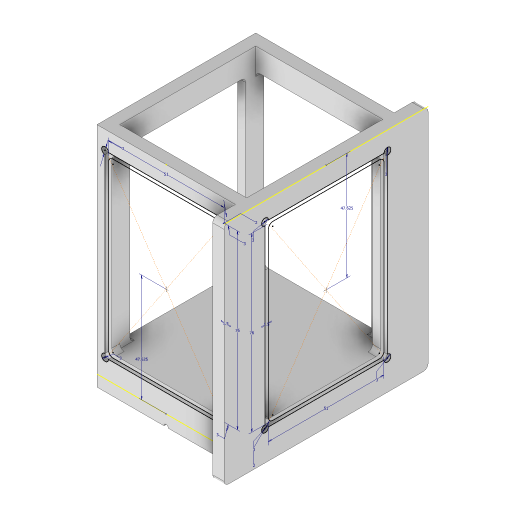
# Autodesk Inventor part: cuvette-w70mm-slide50x75mm-v1
Saved by Autodesk Inventor 2023 (Build 270158000, 158)
## iProperties
Created: 2025-09-30
Part Number: cuvette-w70mm-slide50x75mm-v1
Material: Generic
Document SubType Name: Modeling
Designer: N.Vladimirov
Density: 1 g/cm^3
Appearance: Default
Author: N.Vladimirov
Autodesk Inventor part; units mm, degrees
ref_plane "YZ Plane" through (0, 0, 0) normal (1, 0, 0) x (0, 1, 0)
ref_plane "XZ Plane" through (0, 0, 0) normal (0, 1, 0) x (-1, 0, 0)
ref_plane "XY Plane" through (0, 0, 0) normal (0, 0, 1) x (1, 0, 0)
sketch "Sketch1" plane through (0, 0, 0) normal (0, 0, 1) x (1, 0, 0)
  line L0 (30.5, -35) -> (-30.5, -35)
  line L1 (-30.5, -35) -> (-30.5, 35)
  line L2 (-30.5, 35) -> (30.5, 35)
  line L3 (30.5, 35) -> (30.5, -35)
  line L4 (30.5, -35) -> (-30.5, 35) construction
  line L5 (-30.5, -35) -> (30.5, 35) construction
  point P0 (0, 0)
  dimension "d0" = 61
  dimension "d1" = 70
  constraints: 12 end point, 2 midpoint, 2 parallel, 1 horizontal, 1 perpendicular
  measures "d0" distance of L1.end L2.end
  measures "d1" distance of L0.end L1.end
extrude "Extrusion1" add sketch "Sketch1" along normal blind 95.25
sketch "Sketch2" plane through (30.5, -35, 0) normal (1, 0, 0) x (0, 0, -1)
  line L0 (0, 0) -> (0, 70) projected
  line L1 (0, 70) -> (-95.25, 70) projected
  line L2 (-95.25, 0) -> (-95.25, 70) projected
  line L3 (0, 0) -> (-95.25, 0) projected
  line L4 (0, 70) -> (-95.25, 70) projected
  line L5 (-95.25, 70) -> (0, 70)
  line L6 (0, 70) -> (0, 80)
  line L7 (0, 80) -> (-95.25, 80)
  line L8 (-95.25, 80) -> (-95.25, 70)
  line L9 (-95.25, 70) -> (-95.25, 0) projected
  line L10 (-95.25, 0) -> (0, 0)
  line L11 (0, 0) -> (0, -10)
  line L12 (0, -10) -> (-95.25, -10)
  line L13 (-95.25, -10) -> (-95.25, 0)
  point P0 (0, 35)
  dimension "d4" = 10
  dimension "d5" = 10
  constraints: 16 end point, 4 parallel, 2 horizontal, 2 perpendicular, 1 point on line
  measures "d4" distance of L6.end L5.end
  measures "d5" distance of L10.end L11.end
extrude "Extrusion2" add sketch "Sketch2" along normal blind 5
sketch "Sketch3" plane through (35.5, -35, 0) normal (1, 0, 0) x (0, 0, -1)
  line L0 (0, -10) -> (0, 80) projected
  line L1 (-11.625, 9.5) -> (-83.625, 9.5)
  line L2 (-85.625, 11.5) -> (-85.625, 58.5)
  line L3 (-83.625, 60.5) -> (-11.625, 60.5)
  line L4 (-9.625, 58.5) -> (-9.625, 11.5)
  line L5 (-9.625, 9.5) -> (-85.625, 60.5) construction
  line L6 (-85.625, 9.5) -> (-9.625, 60.5) construction
  line L7 (-9.625, 62) -> (-85.625, 62)
  line L8 (-87.125, 60.5) -> (-87.125, 9.5)
  line L9 (-85.625, 8) -> (-9.625, 8)
  line L10 (-8.125, 9.5) -> (-8.125, 60.5)
  arc A0 (-85.625, 62) -> (-87.125, 60.5) centre (-87.125, 62) ccw
  arc A1 (-8.125, 60.5) -> (-9.625, 62) centre (-8.125, 62) ccw
  arc A2 (-87.125, 9.5) -> (-85.625, 8) centre (-87.125, 8) ccw
  arc A3 (-9.625, 8) -> (-8.125, 9.5) centre (-8.125, 8) ccw
  arc A4 (-83.625, 60.5) -> (-85.625, 58.5) centre (-83.625, 58.5) ccw
  arc A5 (-85.625, 11.5) -> (-83.625, 9.5) centre (-83.625, 11.5) ccw
  arc A6 (-9.625, 58.5) -> (-11.625, 60.5) centre (-11.625, 58.5) ccw
  arc A7 (-11.625, 9.5) -> (-9.625, 11.5) centre (-11.625, 11.5) ccw
  point P0 (0, 35)
  point P1 (-47.625, 35)
  point P2 (0, 35)
  dimension "d8" = 47.625
  dimension "d9" = 76
  dimension "d10" = 51
  dimension "d11" = 1.5
  dimension "d12" = 3
  dimension "d13" = 3
  dimension "d14" = 3
  dimension "d15" = 3
  dimension "d16" = 2
  constraints: 20 end point, 16 point on circle, 8 centre point, 8 point on line, 8 tangent, 4 parallel, 3 equal radius, 3 midpoint, 2 perpendicular, 1 horizontal
  measures "d8" distance of point (0, 35) point (-47.625, 35)
  measures "d9" distance of L5.end L6.end
  measures "d10" distance of L6.start L5.end
  measures "d11" distance between parallel lines of L3 L7
  measures "d12" diameter of A0
  measures "d13" diameter of A1
  measures "d14" diameter of A2
  measures "d15" diameter of A3
  measures "d16" radius of A4
extrude "Extrusion3" cut sketch "Sketch3" against normal through all contours L1 A5 L2 A4 L3 A6 L4 A7
extrude "Extrusion4" cut sketch "Sketch3" against normal blind 1.5 contours L1 A5 L2 A4 L3 A6 L4 A7 | A1 L10 A3 L9 A2 L8 A0 L7
sketch "Sketch4" plane through (-30.5, -35, 0) normal (-1, 0, 0) x (0, 0, 1)
  arc A0 (9.625, 62) -> (8.125, 60.5) centre (8.125, 62) ccw projected
  line L0 (8.125, 60.5) -> (8.125, 9.5) projected
  line L1 (85.625, 62) -> (9.625, 62) projected
  arc A1 (8.125, 9.5) -> (9.625, 8) centre (8.125, 8) ccw projected
  line L2 (9.625, 8) -> (85.625, 8) projected
  arc A2 (85.625, 8) -> (87.125, 9.5) centre (87.125, 8) ccw projected
  line L3 (87.125, 9.5) -> (87.125, 60.5) projected
  arc A3 (87.125, 60.5) -> (85.625, 62) centre (87.125, 62) ccw projected
  point P0 (0, 35)
extrude "Extrusion5" cut sketch "Sketch4" against normal blind 1.5
sketch "Sketch5" plane through (-30.5, 35, 95.25) normal (0, 1, 0) x (1, 0, 0)
  line L0 (61, 0) -> (0, 0) projected
  line L1 (7, 9.625) -> (54, 9.625)
  line L2 (56, 11.625) -> (56, 83.625)
  line L3 (54, 85.625) -> (7, 85.625)
  line L4 (5, 83.625) -> (5, 11.625)
  line L5 (5, 9.625) -> (56, 85.625) construction
  line L6 (56, 9.625) -> (5, 85.625) construction
  line L7 (57.5, 85.625) -> (57.5, 9.625)
  line L8 (56, 8.125) -> (5, 8.125)
  line L9 (3.5, 9.625) -> (3.5, 85.625)
  line L10 (5, 87.125) -> (56, 87.125)
  arc A0 (57.5, 85.625) -> (56, 87.125) centre (57.5, 87.125) ccw
  arc A1 (5, 87.125) -> (3.5, 85.625) centre (3.5, 87.125) ccw
  arc A2 (56, 8.125) -> (57.5, 9.625) centre (57.5, 8.125) ccw
  arc A3 (3.5, 9.625) -> (5, 8.125) centre (3.5, 8.125) ccw
  arc A4 (56, 83.625) -> (54, 85.625) centre (54, 83.625) ccw
  arc A5 (7, 85.625) -> (5, 83.625) centre (7, 83.625) ccw
  arc A6 (54, 9.625) -> (56, 11.625) centre (54, 11.625) ccw
  arc A7 (5, 11.625) -> (7, 9.625) centre (7, 11.625) ccw
  point P0 (30.5, 95.25)
  point P1 (30.5, 47.625)
  point P2 (30.5, 0)
  dimension "d23" = 47.625
  dimension "d24" = 51
  dimension "d25" = 76
  dimension "d26" = 1.5
  dimension "d27" = 3
  dimension "d28" = 3
  dimension "d29" = 3
  dimension "d30" = 3
  dimension "d31" = 2
  constraints: 20 end point, 16 point on circle, 8 centre point, 8 point on line, 8 tangent, 4 parallel, 3 equal radius, 3 midpoint, 2 perpendicular, 1 horizontal
  measures "d23" distance of point (30.5, 0) point (30.5, 47.625)
  measures "d24" distance of L6.end L5.end
  measures "d25" distance of L5.end L6.start
  measures "d26" distance between parallel lines of L2 L7
  measures "d27" diameter of A0
  measures "d28" diameter of A1
  measures "d29" diameter of A2
  measures "d30" diameter of A3
  measures "d31" radius of A4
extrude "Extrusion6" cut sketch "Sketch5" against normal through all contours A7 L4 A5 L3 A4 L2 A6 L1
extrude "Extrusion7" cut sketch "Sketch5" against normal blind 1.5 contours A7 L4 A5 L3 A4 L2 A6 L1 | L7 A2 L8 A3 L9 A1 L10 A0
sketch "Sketch6" plane through (-30.5, -35, 0) normal (0, -1, 0) x (1, 0, 0)
  line L0 (3.5, 85.625) -> (3.5, 9.625) projected
  arc A0 (3.5, 9.625) -> (5, 8.125) centre (3.5, 8.125) ccw projected
  line L1 (5, 8.125) -> (56, 8.125) projected
  arc A1 (56, 8.125) -> (57.5, 9.625) centre (57.5, 8.125) ccw projected
  line L2 (57.5, 9.625) -> (57.5, 85.625) projected
  arc A2 (57.5, 85.625) -> (56, 87.125) centre (57.5, 87.125) ccw projected
  line L3 (56, 87.125) -> (5, 87.125) projected
  arc A3 (5, 87.125) -> (3.5, 85.625) centre (3.5, 87.125) ccw projected
  point P0 (30.5, 0)
extrude "Extrusion8" cut sketch "Sketch6" against normal blind 1.5
sketch "Sketch7" plane through (0, 0, 95.25) normal (0, 0, 1) x (1, 0, 0)
  line L0 (30.5, 35) -> (-30.5, 35) projected
  line L1 (-30.5, 35) -> (-30.5, -35) projected
  line L2 (-30.5, -35) -> (30.5, -35) projected
  line L3 (30.5, -35) -> (30.5, -45) projected
  line L4 (30.5, -45) -> (35.5, -45) projected
  line L5 (35.5, 45) -> (35.5, -45) projected
  line L6 (30.5, 45) -> (35.5, 45) projected
  line L7 (30.5, 45) -> (30.5, 35) projected
  point P0 (0, 0)
extrude "Extrusion9" add sketch "Sketch7" along normal blind 5
sketch "Sketch9" plane through (0, 0, 0) normal (0, 0, -1) x (-1, 0, 0)
  line L0 (30.5, -35) -> (-30.5, -35) projected
  line L1 (30.5, 35) -> (30.5, -35) projected
  line L2 (-30.5, 35) -> (30.5, 35) projected
  line L3 (-35.5, -45) -> (-35.5, 45)
  line L4 (-30.5, -35) -> (-35.5, -35)
  line L5 (-35.5, -45) -> (-35.5, 45) projected
  line L6 (-30.5, 35) -> (-35.5, 35)
  line L7 (-35.5, -35) -> (-35.5, 35)
  line L8 (-35.5, -35) -> (-35.5, 35)
  line L9 (-35.5, -30) -> (-30.5, -30)
  line L10 (-30.5, -30) -> (25.5, -30)
  line L11 (25.5, -30) -> (25.5, 30)
  line L12 (25.5, 30) -> (-30.5, 30)
  line L13 (-30.5, 30) -> (-35.5, 30)
  line L14 (-30.5, -30) -> (-30.5, 30)
  line L15 (-34, -28.5) -> (-34, -25.5) projected
  point P0 (0, 0)
  point P1 (-34, -27)
  dimension "d40" = 5
  constraints: 22 end point, 2 collinear, 2 perpendicular, 2 point on line, 1 parallel, 4 other
  measures "d40" distance between parallel lines of L0 L10
extrude "Extrusion10" cut sketch "Sketch9" against normal up to surface (85.625 mm away) contours L14 L12 L11 L10
fillet "Fillet1" radius 2 4 edges at (33, 45, 0) (33, 45, 100.25) (33, -45, 0) (33, -45, 100.25)
sketch "Sketch10" plane through (0, 0, 100.25) normal (0, 0, 1) x (1, 0, 0)
  point P0 (0, 0)
  point P1 (0, 0)
  constraints: 1 coincident
hole "Hole1" at (0, 0, 100.25) direction (0, 0, -1) diameter 4.9784 depth 10 tip angle 118 thread size "1/4-20 UNC" class "2B" standard "ANSI Unified Screw Threads"
sketch "Sketch11" plane through (-30.5, 35, 0) normal (0, 1, 0) x (1, 0, 0)
  arc A0 (3.5, -85.625) -> (5, -87.125) centre (3.5, -87.125) ccw projected
  line L0 (3.5, -85.625) -> (3.5, -9.625) projected
  arc A1 (5, -8.125) -> (3.5, -9.625) centre (3.5, -8.125) ccw projected
  line L1 (5, -8.125) -> (56, -8.125) projected
  arc A2 (57.5, -9.625) -> (56, -8.125) centre (57.5, -8.125) ccw projected
  line L2 (57.5, -9.625) -> (57.5, -85.625) projected
  arc A3 (56, -87.125) -> (57.5, -85.625) centre (57.5, -87.125) ccw projected
  line L3 (56, -87.125) -> (5, -87.125) projected
  line L4 (61, 0) -> (0, 0) projected
  line L5 (0, 0) -> (0, -100.25) projected
  line L6 (61, -100.25) -> (0, -100.25) projected
  line L7 (61, 0) -> (61, -100.25) projected
  line L8 (0, -100.25) -> (61, -100.25) projected
  circle A4 centre (30.5, -100.25) radius 1
  point P0 (30.5, 0)
  point P1 (29.5, -100.25)
  point P2 (31.5, -100.25)
  dimension "d51" = 2
  constraints: 1 centre point, 1 coincident, 1 midpoint
  measures "d51" diameter of A4
extrude "Extrusion11" cut sketch "Sketch11" against normal through all contours L6 A4 picked at (30.5402, -99.9191)
body "Solid1"
